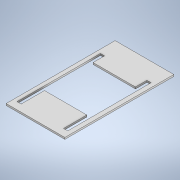
# Autodesk Inventor part: top_part
Saved by Autodesk Inventor 2020 (Build 240168000, 168)
## iProperties
Created: 2019-12-27
Part Number: top_part
Material: Générique
Document SubType Name: Modeling
Designer: damien
Density: 1 g/cm^3
Appearance: Par défaut
Author: damien
Autodesk Inventor part; units mm, degrees
ref_plane "YZ Plane" through (0, 0, 0) normal (1, 0, 0) x (0, 1, 0)
ref_plane "XZ Plane" through (0, 0, 0) normal (0, 1, 0) x (-1, 0, 0)
ref_plane "XY Plane" through (0, 0, 0) normal (0, 0, 1) x (1, 0, 0)
sketch "Esquisse1" plane through (0, 0, 0) normal (0, 1, 0) x (-1, 0, 0)
  line L0 (-350, -650) -> (350, -650)
  line L1 (350, -650) -> (350, 650)
  line L2 (350, 650) -> (-350, 650)
  line L3 (-350, 650) -> (-350, -650)
  line L4 (-350, -650) -> (350, 650) construction
  line L5 (350, -650) -> (-350, 650) construction
  point P0 (0, 0)
  dimension "d0" = 1300
  dimension "d1" = 700
  constraints: 12 end point, 2 midpoint, 2 parallel, 1 horizontal, 1 perpendicular
  measures "d0" distance of L0.end L1.end
  measures "d1" distance of L1.end L2.end
extrude "Extrusion1" add sketch "Esquisse1" along normal blind 20.7
sketch "Esquisse2" plane through (0, 20.7, 0) normal (0, 1, 0) x (1, 0, 0)
  line L0 (-305, -565.5) -> (-305, 429.5)
  line L1 (-305, 429.5) -> (-255, 429.5)
  line L2 (-255, 429.5) -> (-255, 292.5)
  line L3 (-255, 292.5) -> (250, 292.5)
  line L4 (250, 292.5) -> (250, 429.5)
  line L5 (250, 429.5) -> (300, 429.5)
  line L6 (300, 429.5) -> (300, -565.5)
  line L7 (300, -565.5) -> (250, -565.5)
  line L8 (250, -565.5) -> (250, -287.5)
  line L9 (250, -287.5) -> (-255, -287.5)
  line L10 (-255, -287.5) -> (-255, -565.5)
  line L11 (-255, -565.5) -> (-305, -565.5)
  line L12 (350, -650) -> (350, 650) projected
  line L13 (350, 0) -> (300, -68) construction
  line L14 (-350, 650) -> (-350, -650) projected
  line L15 (-350, -650) -> (350, -650) projected
  point P0 (0, 0)
  dimension "d4" = 995
  dimension "d5" = 50
  dimension "d6" = 605
  dimension "d7" = 580
  dimension "d8" = 137
  dimension "d9" = 50
  dimension "d10" = 84.5
  constraints: 26 end point, 7 perpendicular, 6 point on line, 2 equal length, 2 midpoint, 2 vertical
  measures "d4" distance of L5.end L6.end
  measures "d5" distance of L6.end L7.end
  measures "d6" distance between parallel lines of L0 L6
  measures "d7" distance between parallel lines of L3 L9
  measures "d8" distance of L3.end L4.end
  measures "d9" distance between parallel lines of L12 L6
  measures "d10" distance between parallel lines of L15 L11
extrude "Extrusion2" cut sketch "Esquisse2" against normal blind 21.1
